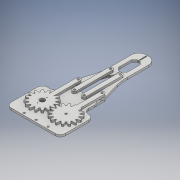
# Autodesk Inventor part: gripper_v3
Saved by Autodesk Inventor 2017 (Build 210142000, 142)
## iProperties
Created: 2016-09-29
Part Number: gripper_v3
Material: Generic
Document SubType Name: Modeling
Designer: mills
Density: 1 g/cm^3
Appearance: Default
Author: mills
Autodesk Inventor part; units mm, degrees
note: some values were not read from the file. Chosen so that the rebuilt part matches the saved one: sketch regions of "Left Gear".
ref_plane "YZ Plane" through (0, 0, 0) normal (1, 0, 0) x (0, 1, 0)
ref_plane "XZ Plane" through (0, 0, 0) normal (0, 1, 0) x (-1, 0, 0)
ref_plane "XY Plane" through (0, 0, 0) normal (0, 0, 1) x (1, 0, 0)
sketch "main drive" plane through (0, 0, 0) normal (0, 0, 1) x (1, 0, 0)
  arc A0 (-24.196, 16.2718) -> (-23.4404, 11.5793) centre (-9.5057, 16.2302) ccw
  arc A1 (-23.4404, 11.5793) -> (-24.5419, 10.8433) centre (-16.5, 0) ccw
  arc A2 (-24.5419, 10.8433) -> (-28.5881, 13.3371) centre (-34.1714, -0.2508) ccw
  arc A3 (-28.5881, 13.3371) -> (-29.8371, 12.0881) centre (-16.5, 0) ccw
  arc A4 (-29.8371, 12.0881) -> (-27.3433, 8.0419) centre (-16.2492, 17.6714) ccw
  arc A5 (-27.3433, 8.0419) -> (-28.0793, 6.9404) centre (-16.5, 0) ccw
  arc A6 (-28.0793, 6.9404) -> (-32.7718, 7.696) centre (-32.7302, -6.9943) ccw
  arc A7 (-32.7718, 7.696) -> (-33.4478, 6.064) centre (-16.5, 0) ccw
  arc A8 (-33.4478, 6.064) -> (-29.5954, 3.2802) centre (-23.0308, 16.4222) ccw
  arc A9 (-29.5954, 3.2802) -> (-29.8539, 1.9809) centre (-16.5, 0) ccw
  arc A10 (-29.8539, 1.9809) -> (-34.4783, 0.8832) centre (-28.8182, -12.6729) ccw
  arc A11 (-34.4783, 0.8832) -> (-34.4783, -0.8832) centre (-16.5, 0) ccw
  arc A12 (-34.4783, -0.8832) -> (-29.8539, -1.9809) centre (-28.8182, 12.6729) ccw
  arc A13 (-29.8539, -1.9809) -> (-29.5954, -3.2802) centre (-16.5, 0) ccw
  arc A14 (-29.5954, -3.2802) -> (-33.4478, -6.064) centre (-23.0308, -16.4222) ccw
  arc A15 (-33.4478, -6.064) -> (-32.7718, -7.696) centre (-16.5, 0) ccw
  arc A16 (-32.7718, -7.696) -> (-28.0793, -6.9404) centre (-32.7302, 6.9943) ccw
  arc A17 (-28.0793, -6.9404) -> (-27.3433, -8.0419) centre (-16.5, 0) ccw
  arc A18 (-27.3433, -8.0419) -> (-29.8371, -12.0881) centre (-16.2492, -17.6714) ccw
  arc A19 (-29.8371, -12.0881) -> (-28.5881, -13.3371) centre (-16.5, 0) ccw
  arc A20 (-28.5881, -13.3371) -> (-24.5419, -10.8433) centre (-34.1714, 0.2508) ccw
  arc A21 (-24.5419, -10.8433) -> (-23.4404, -11.5793) centre (-16.5, 0) ccw
  arc A22 (-23.4404, -11.5793) -> (-24.196, -16.2718) centre (-9.5057, -16.2302) ccw
  arc A23 (-24.196, -16.2718) -> (-22.564, -16.9478) centre (-16.5, 0) ccw
  arc A24 (-22.564, -16.9478) -> (-19.7802, -13.0954) centre (-32.9222, -6.5308) ccw
  arc A25 (-19.7802, -13.0954) -> (-18.4809, -13.3539) centre (-16.5, 0) ccw
  arc A26 (-18.4809, -13.3539) -> (-17.3832, -17.9783) centre (-3.8271, -12.3182) ccw
  arc A27 (-17.3832, -17.9783) -> (-15.6168, -17.9783) centre (-16.5, 0) ccw
  arc A28 (-15.6168, -17.9783) -> (-14.5191, -13.3539) centre (-29.1729, -12.3182) ccw
  arc A29 (-14.5191, -13.3539) -> (-13.2198, -13.0954) centre (-16.5, 0) ccw
  arc A30 (-13.2198, -13.0954) -> (-10.436, -16.9478) centre (-0.0778, -6.5308) ccw
  arc A31 (-10.436, -16.9478) -> (-8.804, -16.2718) centre (-16.5, 0) ccw
  arc A32 (-8.804, -16.2718) -> (-9.5596, -11.5793) centre (-23.4943, -16.2302) ccw
  arc A33 (-9.5596, -11.5793) -> (-8.4581, -10.8433) centre (-16.5, 0) ccw
  arc A34 (-8.4581, -10.8433) -> (-4.4119, -13.3371) centre (1.1714, 0.2508) ccw
  arc A35 (-4.4119, -13.3371) -> (-3.1629, -12.0881) centre (-16.5, 0) ccw
  arc A36 (-3.1629, -12.0881) -> (-5.6567, -8.0419) centre (-16.7508, -17.6714) ccw
  arc A37 (-5.6567, -8.0419) -> (-4.9207, -6.9404) centre (-16.5, 0) ccw
  arc A38 (-4.9207, -6.9404) -> (-0.2282, -7.696) centre (-0.2698, 6.9943) ccw
  arc A39 (-0.2282, -7.696) -> (0.4478, -6.064) centre (-16.5, 0) ccw
  arc A40 (0.4478, -6.064) -> (-3.4046, -3.2802) centre (-9.9692, -16.4222) ccw
  arc A41 (-3.4046, -3.2802) -> (-3.1461, -1.9809) centre (-16.5, 0) ccw
  arc A42 (-3.1461, -1.9809) -> (1.4783, -0.8832) centre (-4.1818, 12.6729) ccw
  arc A43 (1.4783, -0.8832) -> (1.4783, 0.8832) centre (-16.5, 0) ccw
  arc A44 (1.4783, 0.8832) -> (-3.1461, 1.9809) centre (-4.1818, -12.6729) ccw
  arc A45 (-3.1461, 1.9809) -> (-3.4046, 3.2802) centre (-16.5, 0) ccw
  arc A46 (-3.4046, 3.2802) -> (0.4478, 6.064) centre (-9.9692, 16.4222) ccw
  arc A47 (0.4478, 6.064) -> (-0.2282, 7.696) centre (-16.5, 0) ccw
  arc A48 (-0.2282, 7.696) -> (-4.9207, 6.9404) centre (-0.2698, -6.9943) ccw
  arc A49 (-4.9207, 6.9404) -> (-5.6567, 8.0419) centre (-16.5, 0) ccw
  arc A50 (-5.6567, 8.0419) -> (-3.1629, 12.0881) centre (-16.7508, 17.6714) ccw
  arc A51 (-3.1629, 12.0881) -> (-4.4119, 13.3371) centre (-16.5, 0) ccw
  arc A52 (-4.4119, 13.3371) -> (-8.4581, 10.8433) centre (1.1714, -0.2508) ccw
  arc A53 (-8.4581, 10.8433) -> (-9.5596, 11.5793) centre (-16.5, 0) ccw
  arc A54 (-9.5596, 11.5793) -> (-8.804, 16.2718) centre (-23.4943, 16.2302) ccw
  arc A55 (-8.804, 16.2718) -> (-10.436, 16.9478) centre (-16.5, 0) ccw
  arc A56 (-10.436, 16.9478) -> (-13.2198, 13.0954) centre (-0.0778, 6.5308) ccw
  arc A57 (-13.2198, 13.0954) -> (-14.5191, 13.3539) centre (-16.5, 0) ccw
  arc A58 (-14.5191, 13.3539) -> (-15.6168, 17.9783) centre (-29.1729, 12.3182) ccw
  arc A59 (-15.6168, 17.9783) -> (-17.3832, 17.9783) centre (-16.5, 0) ccw
  arc A60 (-17.3832, 17.9783) -> (-18.4809, 13.3539) centre (-3.8271, 12.3182) ccw
  arc A61 (-18.4809, 13.3539) -> (-19.7802, 13.0954) centre (-16.5, 0) ccw
  arc A62 (-19.7802, 13.0954) -> (-22.564, 16.9478) centre (-32.9222, 6.5308) ccw
  arc A63 (-22.564, 16.9478) -> (-24.196, 16.2718) centre (-16.5, 0) ccw
  arc A64 (5.8406, 14.5044) -> (7.4777, 10.0423) centre (20.2689, 17.2666) ccw
  arc A65 (7.4777, 10.0423) -> (6.5368, 9.1096) centre (16.5, 0) ccw
  arc A66 (6.5368, 9.1096) -> (2.0892, 10.7856) centre (-0.7989, -3.6181) ccw
  arc A67 (2.0892, 10.7856) -> (1.1014, 9.3211) centre (16.5, 0) ccw
  arc A68 (1.1014, 9.3211) -> (4.3214, 5.8252) centre (13.3744, 17.3946) ccw
  arc A69 (4.3214, 5.8252) -> (3.8091, 4.6034) centre (16.5, 0) ccw
  arc A70 (3.8091, 4.6034) -> (-0.9413, 4.4498) centre (1.9025, -9.9627) ccw
  arc A71 (-0.9413, 4.4498) -> (-1.2935, 2.7188) centre (16.5, 0) ccw
  arc A72 (-1.2935, 2.7188) -> (3.0193, 0.7212) centre (6.9557, 14.8744) ccw
  arc A73 (3.0193, 0.7212) -> (3.0135, -0.6036) centre (16.5, 0) ccw
  arc A74 (3.0135, -0.6036) -> (-1.3165, -2.5634) centre (6.8262, -14.7905) ccw
  arc A75 (-1.3165, -2.5634) -> (-0.9795, -4.2974) centre (16.5, 0) ccw
  arc A76 (-0.9795, -4.2974) -> (3.7694, -4.4925) centre (1.99, 10.0897) ccw
  arc A77 (3.7694, -4.4925) -> (4.2711, -5.7187) centre (16.5, 0) ccw
  arc A78 (4.2711, -5.7187) -> (1.0206, -9.1864) centre (13.2227, -17.3666) ccw
  arc A79 (1.0206, -9.1864) -> (1.9956, -10.6594) centre (16.5, 0) ccw
  arc A80 (1.9956, -10.6594) -> (6.4577, -9.0223) centre (-0.7666, 3.7689) ccw
  arc A81 (6.4577, -9.0223) -> (7.3904, -9.9632) centre (16.5, 0) ccw
  arc A82 (7.3904, -9.9632) -> (5.7144, -14.4108) centre (20.1181, -17.2988) ccw
  arc A83 (5.7144, -14.4108) -> (7.1789, -15.3986) centre (16.5, 0) ccw
  arc A84 (7.1789, -15.3986) -> (10.6748, -12.1786) centre (-0.8946, -3.1256) ccw
  arc A85 (10.6748, -12.1786) -> (11.8966, -12.6909) centre (16.5, 0) ccw
  arc A86 (11.8966, -12.6909) -> (12.0502, -17.4413) centre (26.4627, -14.5975) ccw
  arc A87 (12.0502, -17.4413) -> (13.7812, -17.7935) centre (16.5, 0) ccw
  arc A88 (13.7812, -17.7935) -> (15.7788, -13.4807) centre (1.6256, -9.5443) ccw
  arc A89 (15.7788, -13.4807) -> (17.1036, -13.4865) centre (16.5, 0) ccw
  arc A90 (17.1036, -13.4865) -> (19.0634, -17.8165) centre (31.2905, -9.6737) ccw
  arc A91 (19.0634, -17.8165) -> (20.7974, -17.4795) centre (16.5, 0) ccw
  arc A92 (20.7974, -17.4795) -> (20.9925, -12.7306) centre (6.4103, -14.51) ccw
  arc A93 (20.9925, -12.7306) -> (22.2187, -12.2289) centre (16.5, 0) ccw
  arc A94 (22.2187, -12.2289) -> (25.6864, -15.4793) centre (33.8666, -3.2773) ccw
  arc A95 (25.6864, -15.4793) -> (27.1594, -14.5044) centre (16.5, 0) ccw
  arc A96 (27.1594, -14.5044) -> (25.5223, -10.0423) centre (12.7311, -17.2666) ccw
  arc A97 (25.5223, -10.0423) -> (26.4632, -9.1096) centre (16.5, 0) ccw
  arc A98 (26.4632, -9.1096) -> (30.9108, -10.7856) centre (33.7988, 3.6181) ccw
  arc A99 (30.9108, -10.7856) -> (31.8986, -9.3211) centre (16.5, 0) ccw
  arc A100 (31.8986, -9.3211) -> (28.6786, -5.8252) centre (19.6256, -17.3946) ccw
  arc A101 (28.6786, -5.8252) -> (29.1909, -4.6034) centre (16.5, 0) ccw
  arc A102 (29.1909, -4.6034) -> (33.9413, -4.4498) centre (31.0975, 9.9627) ccw
  arc A103 (33.9413, -4.4498) -> (34.2935, -2.7188) centre (16.5, 0) ccw
  arc A104 (34.2935, -2.7188) -> (29.9807, -0.7212) centre (26.0443, -14.8744) ccw
  arc A105 (29.9807, -0.7212) -> (29.9865, 0.6036) centre (16.5, 0) ccw
  arc A106 (29.9865, 0.6036) -> (34.3165, 2.5634) centre (26.1738, 14.7905) ccw
  arc A107 (34.3165, 2.5634) -> (33.9795, 4.2974) centre (16.5, 0) ccw
  arc A108 (33.9795, 4.2974) -> (29.2306, 4.4925) centre (31.01, -10.0897) ccw
  arc A109 (29.2306, 4.4925) -> (28.7289, 5.7187) centre (16.5, 0) ccw
  arc A110 (28.7289, 5.7187) -> (31.9794, 9.1864) centre (19.7773, 17.3666) ccw
  arc A111 (31.9794, 9.1864) -> (31.0044, 10.6594) centre (16.5, 0) ccw
  arc A112 (31.0044, 10.6594) -> (26.5423, 9.0223) centre (33.7666, -3.7689) ccw
  arc A113 (26.5423, 9.0223) -> (25.6096, 9.9632) centre (16.5, 0) ccw
  arc A114 (25.6096, 9.9632) -> (27.2856, 14.4108) centre (12.8819, 17.2989) ccw
  arc A115 (27.2856, 14.4108) -> (25.8211, 15.3986) centre (16.5, 0) ccw
  arc A116 (25.8211, 15.3986) -> (22.3252, 12.1786) centre (33.8946, 3.1256) ccw
  arc A117 (22.3252, 12.1786) -> (21.1034, 12.6909) centre (16.5, 0) ccw
  arc A118 (21.1034, 12.6909) -> (20.9498, 17.4413) centre (6.5373, 14.5975) ccw
  arc A119 (20.9498, 17.4413) -> (19.2188, 17.7935) centre (16.5, 0) ccw
  arc A120 (19.2188, 17.7935) -> (17.2212, 13.4807) centre (31.3744, 9.5443) ccw
  arc A121 (17.2212, 13.4807) -> (15.8964, 13.4865) centre (16.5, 0) ccw
  arc A122 (15.8964, 13.4865) -> (13.9366, 17.8165) centre (1.7095, 9.6738) ccw
  arc A123 (13.9366, 17.8165) -> (12.2026, 17.4795) centre (16.5, 0) ccw
  arc A124 (12.2026, 17.4795) -> (12.0075, 12.7306) centre (26.5897, 14.51) ccw
  arc A125 (12.0075, 12.7306) -> (10.7813, 12.2289) centre (16.5, 0) ccw
  arc A126 (10.7813, 12.2289) -> (7.3136, 15.4794) centre (-0.8666, 3.2773) ccw
  arc A127 (7.3136, 15.4794) -> (5.8406, 14.5044) centre (16.5, 0) ccw
  circle A128 centre (16.5, 0) radius 1.375
  circle A129 centre (-16.5, 6.5) radius 0.5
  circle A130 centre (-16.5, -6.5) radius 0.5
  line L0 (-16.5, 111.9513) -> (-16.5, -38.0487) construction
  line L1 (16.5, 111.9513) -> (16.5, -38.0487) construction
  line L2 (19.5, 50) -> (19.5, 0)
  line L3 (13.5, 0) -> (13.5, 50)
  circle A131 centre (16.5, 50) radius 1.375
  circle A132 centre (16.5, 50) radius 3
  line L4 (13.5, 50) -> (15.125, 50)
  line L5 (17.875, 50) -> (19.5, 50)
  line L6 (19.5, 0) -> (17.875, 0)
  line L7 (15.125, 0) -> (13.5, 0)
  line L8 (-48.3069, 0) -> (48.1802, 0) projected
  line L9 (-3.75, 85) -> (-3.75, 35)
  line L10 (-9.75, 35) -> (-9.75, 85)
  line L11 (9.75, 85) -> (9.75, 35)
  line L12 (3.75, 35) -> (3.75, 85)
  line L13 (-6.75, 111.9513) -> (-6.75, -38.0487) construction
  line L14 (6.75, 111.9513) -> (6.75, -38.0487) construction
  line L15 (0, -68.0487) -> (0, 141.9513) projected
  line L16 (-19.5, 0) -> (-13.5, 0)
  line L17 (-13.5, 0) -> (-13.5, 50)
  line L18 (-19.5, 50) -> (-19.5, 0)
  circle A133 centre (-16.5, 50) radius 3
  circle A134 centre (-16.5, 0) radius 3.45
  circle A135 centre (-16.5, 50) radius 1.375
  line L19 (-13.5, 50) -> (-15.125, 50)
  line L20 (-17.875, 50) -> (-19.5, 50)
  circle A136 centre (-6.75, 85) radius 3
  circle A137 centre (6.75, 85) radius 3
  circle A138 centre (6.75, 35) radius 3
  circle A139 centre (-6.75, 35) radius 3
  circle A140 centre (-6.75, 35) radius 1.375
  circle A141 centre (6.75, 35) radius 1.375
  circle A142 centre (6.75, 85) radius 1.375
  circle A143 centre (-6.75, 85) radius 1.375
  line L21 (-3.75, 35) -> (-5.375, 35)
  line L22 (-8.125, 35) -> (-9.75, 35)
  line L23 (9.75, 35) -> (8.125, 35)
  line L24 (5.375, 35) -> (3.75, 35)
  line L25 (3.75, 85) -> (5.375, 85)
  line L26 (8.125, 85) -> (9.75, 85)
  line L27 (-9.75, 85) -> (-8.125, 85)
  line L28 (-5.375, 85) -> (-3.75, 85)
  point P0 (0, 0)
  dimension "d15" = 2.75
  dimension "d12" = 16.5
  dimension "d13" = 16.5
  dimension "d16" = 1
  dimension "d17" = 1
  dimension "d18" = 13
  dimension "d31" = 50
  dimension "d35" = 6
  dimension "d36" = 6
  dimension "d37" = 3
  dimension "d38" = 3
  dimension "d44" = 3.75
  dimension "d46" = 3.75
  dimension "d47" = 50
  dimension "d50" = 6.5
  dimension "d51" = 50
  dimension "d52" = 6
  dimension "d53" = 6
  dimension "d54" = 3
  dimension "d55" = 3
  dimension "d56" = 6.9
  dimension "d57" = 2.75
  dimension "d58" = 2.75
  dimension "d63" = 2.75
  dimension "d64" = 2.75
  dimension "d65" = 2.75
  dimension "d66" = 2.75
  constraints: 140 point on circle, 73 centre point, 62 equal radius, 54 end point, 18 parallel, 9 horizontal alignment, 8 point on line, 8 vertical, 7 horizontal, 7 perpendicular, 6 coincident, 2 collinear, 2 vertical alignment, 203 other
  measures "d16" diameter of A129
  measures "d17" diameter of A130
  measures "d18" distance of A130.centre A129.centre
  measures "d31" distance of L2.start L2.end
  measures "d35" distance of L10.end L9.start
  measures "d36" distance of L12.end L11.start
  measures "d37" distance between parallel lines of L13 L10
  measures "d38" distance between parallel lines of L14 L11
  measures "d44" distance between parallel lines of L15 L9
  measures "d46" distance between parallel lines of L12 L15
  measures "d47" distance of L11.start L11.end
  measures "d51" distance of L18.start L16.start
  measures "d52" distance of L17.end L18.start
  measures "d53" distance between parallel lines of L2 L3
  measures "d54" distance between parallel lines of L3 L1
  measures "d55" distance between parallel lines of L17 L0
  measures "d56" diameter of A134
  measures "d57" diameter of A135
  measures "d58" diameter of A131
  measures "d63" diameter of A143
  measures "d64" diameter of A140
  measures "d65" diameter of A141
  measures "d66" diameter of A142
extrude "Left Gear" add sketch "main drive" along normal blind 3 contours A63 A62 A61 L18 A134 L8 A11 A10 A9 A8 A7 A6 A5 A4 A3 A2 A1 A0 | L18 A133 L17 A57 A58 A59 A60 A61 | A61 A60 A59 A58 A57 L17 A134 L18 | L20 A135 L19 A133 | A133 L19 A135 L20 | L17 A57 A56 A55 A54 A53 A52 A51 A50 A49 A48 A47 L15 A46 A45 A44 L8 A134 | A134 L8 L15 A42 A41 A40 A39 A38 A37 A36 A35 A34 A33 A32 A31 A30 A29 A28 A27 A26 A25 A24 A23 A22 A21 A20 A19 A18 A17 A16 A15 A14 A13 A12 A11 | L15 A44 A43 L8 | L8 A43 A42 L15 | A40 A39 L15 | L15 A47 A46
extrude "Left Gear cutout" cut sketch "main drive" along normal blind 3 contours A134 L17 L8 L18 | L18 L8 A134 | L8 A134 | A134 L8 L17
extrude "Right Gear" add sketch "main drive" along normal blind 3 separate body contours L8 L7 A128 L6 A105 A104 A103 A102 A101 A100 A99 A98 A97 A96 A95 A94 A93 A92 A91 A90 A89 A88 A87 A86 A85 A84 A83 A82 A81 A80 A79 A78 A77 A76 L15 A74 A73 | A73 A72 L15 A70 A69 A68 A67 A66 A65 A64 A127 A126 A125 A124 A123 L3 L8 | L15 A76 A75 A74 | A72 A71 A70 L15 | L3 A123 A122 A121 A120 A119 L2 L6 A128 L7 | L3 A132 L2 A119 A120 A121 A122 A123 | L4 A131 L5 A132 | A132 L5 A131 L4 | L2 A119 A118 A117 A116 A115 A114 A113 A112 A111 A110 A109 A108 A107 A106 A105 L8
extrude "Left Strut" add sketch "main drive" along normal blind 3 separate body contours L28 A143 L27 A136 | L9 A139 L10 A136 | A136 L27 A143 L28 | L21 A140 L22 A139 | A139 L22 A140 L21
extrude "Right Strut" add sketch "main drive" along normal blind 3 separate body contours L26 A142 L25 A137 | L11 A138 L12 A137 | A137 L25 A142 L26 | L23 A141 L24 A138 | A138 L24 A141 L23
sketch "grip + base" plane through (0, 0, 0) normal (0, 0, -1) x (-1, 0, 0)
  line L0 (4.0208, 79.5) -> (12.0208, 79.5)
  line L1 (12.0208, 89.186) -> (12.0208, 119.3579)
  line L2 (1.8786, 129.5) -> (0.0208, 129.5)
  line L3 (0.0208, 129.5) -> (0.0208, 83.5)
  line L4 (0.0208, 117.5) -> (2.0208, 117.5)
  line L5 (6.0208, 113.5) -> (6.0208, 95.5)
  line L6 (2.0208, 91.5) -> (0.0208, 91.5)
  line L7 (0.0208, 91.5) -> (0.0208, 117.5)
  line L8 (2.0208, 117.5) -> (6.0208, 113.5)
  line L9 (6.0208, 95.5) -> (2.0208, 91.5)
  line L10 (8.9497, 126.5711) -> (9.0918, 126.4289)
  line L11 (0.0208, 128.2) -> (0.8868, 127.7)
  line L12 (0.8868, 127.7) -> (0.0208, 127.2)
  line L13 (0.0208, 128.2) -> (0.0208, 127.2)
  line L14 (0.0208, 127) -> (0.8868, 126.5)
  line L15 (0.0208, 127) -> (0.0208, 126)
  line L16 (0.8868, 126.5) -> (0.0208, 126)
  line L17 (0.0208, 125.8) -> (0.8868, 125.3)
  line L18 (0.0208, 125.8) -> (0.0208, 124.8)
  line L19 (0.8868, 125.3) -> (0.0208, 124.8)
  line L20 (0.0208, 124.6) -> (0.8868, 124.1)
  line L21 (0.0208, 124.6) -> (0.0208, 123.6)
  line L22 (0.8868, 124.1) -> (0.0208, 123.6)
  line L23 (0.0208, 123.4) -> (0.8868, 122.9)
  line L24 (0.0208, 123.4) -> (0.0208, 122.4)
  line L25 (0.8868, 122.9) -> (0.0208, 122.4)
  line L26 (0.0208, 122.2) -> (0.8868, 121.7)
  line L27 (0.0208, 122.2) -> (0.0208, 121.2)
  line L28 (0.8868, 121.7) -> (0.0208, 121.2)
  line L29 (0.0208, 121) -> (0.8868, 120.5)
  line L30 (0.0208, 121) -> (0.0208, 120)
  line L31 (0.8868, 120.5) -> (0.0208, 120)
  line L32 (0.0208, 119.8) -> (0.8868, 119.3)
  line L33 (0.0208, 119.8) -> (0.0208, 118.8)
  line L34 (0.8868, 119.3) -> (0.0208, 118.8)
  line L35 (6.75, 85) -> (16.5, 50) construction
  line L36 (4.7706, 77.1999) -> (12.6467, 48.9266)
  line L37 (20.3533, 51.0734) -> (14.2215, 73.0848)
  arc A0 (10.6033, 86.0734) -> (2.8967, 83.9266) centre (6.75, 85) ccw
  arc A1 (12.6467, 48.9266) -> (20.3533, 51.0734) centre (16.5, 50) ccw
  arc A2 (12.0208, 89.186) -> (14.2215, 73.0848) centre (72.0208, 89.186) ccw
  arc A3 (12.0208, 119.3579) -> (9.0918, 126.4289) centre (2.0208, 119.3579) ccw
  arc A4 (8.9497, 126.5711) -> (1.8786, 129.5) centre (1.8786, 119.5) ccw
  line L38 (12.0208, 79.5) -> (12.8078, 79.5)
  arc A5 (0.0208, 83.5) -> (2.469, 79.8133) centre (4.0208, 83.5) ccw
  arc A6 (4.7706, 77.1999) -> (2.469, 79.8133) centre (0.9173, 76.1265) ccw
  circle A7 centre (6.75, 85) radius 1.375 projected
  circle A8 centre (16.5, 50) radius 1.375 projected
  line L39 (0, -47.6407) -> (0, 159.8439) projected
  line L40 (-4.0208, 79.5) -> (-12.0208, 79.5)
  line L41 (-12.0208, 89.186) -> (-12.0208, 119.3579)
  line L42 (-1.8786, 129.5) -> (-0.0208, 129.5)
  line L43 (-0.0208, 129.5) -> (-0.0208, 83.5)
  line L44 (-0.0208, 117.5) -> (-2.0208, 117.5)
  line L45 (-6.0208, 113.5) -> (-6.0208, 95.5)
  line L46 (-2.0208, 91.5) -> (-0.0208, 91.5)
  line L47 (-0.0208, 91.5) -> (-0.0208, 117.5)
  line L48 (-2.0208, 117.5) -> (-6.0208, 113.5)
  line L49 (-6.0208, 95.5) -> (-2.0208, 91.5)
  line L50 (-8.9497, 126.5711) -> (-9.0918, 126.4289)
  line L51 (-0.0208, 128.2) -> (-0.8868, 127.7)
  line L52 (-0.8868, 127.7) -> (-0.0208, 127.2)
  line L53 (-0.0208, 128.2) -> (-0.0208, 127.2)
  line L54 (-0.0208, 127) -> (-0.8868, 126.5)
  line L55 (-0.0208, 127) -> (-0.0208, 126)
  line L56 (-0.8868, 126.5) -> (-0.0208, 126)
  line L57 (-0.0208, 125.8) -> (-0.8868, 125.3)
  line L58 (-0.0208, 125.8) -> (-0.0208, 124.8)
  line L59 (-0.8868, 125.3) -> (-0.0208, 124.8)
  line L60 (-0.0208, 124.6) -> (-0.8868, 124.1)
  line L61 (-0.0208, 124.6) -> (-0.0208, 123.6)
  line L62 (-0.8868, 124.1) -> (-0.0208, 123.6)
  line L63 (-0.0208, 123.4) -> (-0.8868, 122.9)
  line L64 (-0.0208, 123.4) -> (-0.0208, 122.4)
  line L65 (-0.8868, 122.9) -> (-0.0208, 122.4)
  line L66 (-0.0208, 122.2) -> (-0.8868, 121.7)
  line L67 (-0.0208, 122.2) -> (-0.0208, 121.2)
  line L68 (-0.8868, 121.7) -> (-0.0208, 121.2)
  line L69 (-0.0208, 121) -> (-0.8868, 120.5)
  line L70 (-0.0208, 121) -> (-0.0208, 120)
  line L71 (-0.8868, 120.5) -> (-0.0208, 120)
  line L72 (-0.0208, 119.8) -> (-0.8868, 119.3)
  line L73 (-0.0208, 119.8) -> (-0.0208, 118.8)
  line L74 (-0.8868, 119.3) -> (-0.0208, 118.8)
  line L75 (-6.75, 85) -> (-16.5, 50) construction
  line L76 (-4.7706, 77.1999) -> (-12.6467, 48.9266)
  line L77 (-20.3533, 51.0734) -> (-14.2215, 73.0848)
  arc A9 (-2.8967, 83.9266) -> (-10.6033, 86.0734) centre (-6.75, 85) ccw
  arc A10 (-20.3533, 51.0734) -> (-12.6467, 48.9266) centre (-16.5, 50) ccw
  arc A11 (-14.2215, 73.0848) -> (-12.0208, 89.186) centre (-72.0208, 89.186) ccw
  arc A12 (-9.0918, 126.4289) -> (-12.0208, 119.3579) centre (-2.0208, 119.3579) ccw
  arc A13 (-1.8786, 129.5) -> (-8.9497, 126.5711) centre (-1.8786, 119.5) ccw
  line L78 (-12.0208, 79.5) -> (-12.8078, 79.5)
  arc A14 (-2.469, 79.8133) -> (-0.0208, 83.5) centre (-4.0208, 83.5) ccw
  arc A15 (-2.469, 79.8133) -> (-4.7706, 77.1999) centre (-0.9173, 76.1265) ccw
  circle A16 centre (-6.75, 85) radius 1.375
  circle A17 centre (-16.5, 50) radius 1.375
  point P0 (0, 0)
  point P1 (12.0208, 129.5)
  point P2 (-6.75, 85)
  point P3 (6.0208, 91.5)
  point P4 (6.0208, 117.5)
  point P5 (6.0208, 129.5)
  point P6 (12.0208, 123.5)
  point P7 (-16.5, 50)
  point P8 (11.625, 67.5)
  point P9 (-12.0208, 129.5)
  point P10 (6.75, 85)
  point P11 (-6.0208, 91.5)
  point P12 (-6.0208, 117.5)
  point P13 (-6.0208, 129.5)
  point P14 (-12.0208, 123.5)
  point P15 (16.5, 50)
  point P16 (-11.625, 67.5)
  dimension "d73" = 12
  dimension "d74" = 50
  dimension "d75" = 5.5
  dimension "d76" = 6
  dimension "d77" = 12
  dimension "d78" = 12
  dimension "d79" = 4
  dimension "d80" = 4
  dimension "d81" = 4
  dimension "d82" = 4
  dimension "d83" = 6
  dimension "d84" = 6
  dimension "d86" = 1
  dimension "d87" = 1
  dimension "d88" = 1
  dimension "d91" = 1.2
  dimension "d96" = 1.3
  dimension "d97" = 9.4
  dimension "d98" = 8
  dimension "d99" = 60
  dimension "d100" = 10
  dimension "d101" = 10
  dimension "d102" = 4
  dimension "d103" = 4
  constraints: 160 end point, 64 symmetric about line, 32 point on circle, 32 point on line, 16 centre point, 14 tangent, 5 parallel, 3 horizontal, 2 perpendicular, 1 collinear, 1 midpoint, 1 vertical, 51 other
  measures "d73" distance of point (12.021, 129.5) L2.end
  measures "d74" distance of L0.end point (12.021, 129.5)
  measures "d75" distance from line of L0 L35.start
  measures "d76" distance of L4.start point (6.021, 117.5)
  measures "d77" distance between parallel lines of L4 L2
  measures "d78" distance between parallel lines of L6 L0
  measures "d79" distance of L4.end point (6.021, 117.5)
  measures "d80" distance of L5.start point (6.021, 117.5)
  measures "d81" distance of L5.end point (6.021, 91.5)
  measures "d82" distance of L6.start point (6.021, 91.5)
  measures "d83" distance of point (6.021, 129.5) point (12.021, 129.5)
  measures "d84" distance of point (12.021, 123.5) point (12.021, 129.5)
  measures "d86" distance of L11.end L12.end
  measures "d87" distance of L11.start L11.end
  measures "d88" distance of L12.end L11.start
  measures "d91" distance of L11.start L14.start
  measures "d96" distance of L2.end L11.start
  measures "d97" distance of L33.end L11.start
  measures "d98" distance between parallel lines of L37 L36
  measures "d99" radius of A2
  measures "d100" radius of A3
  measures "d101" radius of A4
  measures "d102" radius of A5
  measures "d103" radius of A6
extrude "Left Clamp" add sketch "grip + base" along normal blind 3 separate body contours A2 L37 A1 L36 A6 A5 L3 L6 L9 L5 L8 L4 L34 L32 L31 L29 L28 L26 L25 L23 L22 L20 L19 L17 L16 L14 L12 L11 L2 A4 L10 A3 L1
extrude "Right Clamp" add sketch "grip + base" along normal blind 3 separate body contours L41 A12 L50 A13 L42 L43 L51 L52 L54 L56 L57 L59 L60 L62 L63 L65 L66 L68 L69 L71 L72 L74 L44 L48 L45 L49 L46 A14 A15 L76 A10 L77 A11
sketch "Base Sktch" plane through (0, 0, 0) normal (0, 0, -1) x (-1, 0, 0)
  line L0 (13.5, 40) -> (-15.5, 40)
  line L1 (-36.5115, 11) -> (-36.5115, -21)
  line L2 (-29.5115, -28) -> (31.4938, -28)
  line L3 (38.4938, -21) -> (38.4938, 15)
  line L4 (16.5, 111.9513) -> (16.5, -38.0487) construction
  line L5 (-16.5, 111.9513) -> (-16.5, -38.0487) construction
  arc A0 (20.5, 33) -> (13.5, 40) centre (13.5, 33) ccw
  arc A1 (-15.5, 40) -> (-22.5, 33) centre (-15.5, 33) ccw
  line L6 (48.3069, 0) -> (-48.1802, 0) projected
  line L7 (31.4938, 22) -> (27.5, 22)
  line L8 (-29.5, 18) -> (-29.5115, 18)
  line L9 (20.5, 29) -> (20.5, 33)
  line L10 (-22.5, 33) -> (-22.5, 25)
  arc A2 (20.5, 29) -> (27.5, 22) centre (27.5, 29) ccw
  arc A3 (38.4938, 15) -> (31.4938, 22) centre (31.4938, 15) ccw
  arc A4 (-29.5, 18) -> (-22.5, 25) centre (-29.5, 25) ccw
  arc A5 (-29.5115, 18) -> (-36.5115, 11) centre (-29.5115, 11) ccw
  line L11 (22.375, 16.6) -> (10.625, 16.6)
  line L12 (10.625, 16.6) -> (10.625, -5.8)
  line L13 (10.625, -5.8) -> (22.375, -5.8)
  line L14 (22.375, -5.8) -> (22.375, 16.6)
  line L15 (7.625, 21.6) -> (25.375, 21.6)
  line L16 (25.375, 21.6) -> (25.375, -10.8)
  line L17 (25.375, -10.8) -> (7.625, -10.8)
  line L18 (7.625, -10.8) -> (7.625, 21.6)
  circle A6 centre (16.5, 18.85) radius 1
  circle A7 centre (16.5, -8.05) radius 1
  circle A8 centre (-16.5, -25) radius 1.375
  circle A9 centre (0, -25) radius 1.375
  circle A10 centre (16.5, -25) radius 1.375
  arc A11 (-36.5115, -21) -> (-29.5115, -28) centre (-29.5115, -21) ccw
  arc A12 (31.4938, -28) -> (38.4938, -21) centre (31.4938, -21) ccw
  circle A13 centre (-16.5, 0) radius 1.375 projected
  circle A14 centre (-6.75, 35) radius 1.375 projected
  circle A15 centre (6.75, 35) radius 1.375 projected
  point P0 (0, 0)
  point P1 (16.5, 22)
  point P2 (-16.5, 18)
  point P3 (20.5, 0)
  point P4 (-22.5, 0)
  point P5 (16.5, 0)
  dimension "d116" = 5
  dimension "d119" = 7
  dimension "d122" = 28
  dimension "d123" = 7
  dimension "d125" = 11.75
  dimension "d126" = 22.4
  dimension "d128" = 5.875
  dimension "d129" = 17.75
  dimension "d130" = 32.4
  dimension "d133" = 8.875
  dimension "d135" = 5
  dimension "d136" = 2
  dimension "d137" = 2
  dimension "d138" = 2.25
  dimension "d139" = 2.25
  dimension "d140" = 2.75
  dimension "d141" = 2.75
  dimension "d142" = 2.75
  dimension "d143" = 3
  dimension "d144" = 3
  dimension "d145" = 3
  dimension "d146" = 7
  dimension "d161" = 5.8
  constraints: 32 end point, 16 point on circle, 16 tangent, 14 point on line, 13 centre point, 8 parallel, 5 equal radius, 5 horizontal, 5 perpendicular
  measures "d116" distance from line of L0 point (6.75, 35)
  measures "d119" radius of A0
  measures "d122" distance between parallel lines of L6 L2
  measures "d123" radius of A2
  measures "d125" distance of L12.end L13.end
  measures "d126" distance of L13.end L11.start
  measures "d128" distance from line of L14 point (16.5, 0)
  measures "d129" distance of L15.start L15.end
  measures "d130" distance of L15.end L16.end
  measures "d133" distance between parallel lines of L4 L18
  measures "d135" distance between parallel lines of L15 L11
  measures "d136" diameter of A6
  measures "d137" diameter of A7
  measures "d138" distance from line of A6.centre L11
  measures "d139" distance from line of L13 A7.centre
  measures "d140" diameter of A8
  measures "d141" diameter of A9
  measures "d142" diameter of A10
  measures "d143" distance from line of L2 A8.centre
  measures "d144" distance from line of L2 A9.centre
  measures "d145" distance from line of L2 A10.centre
  measures "d146" radius of A11
  measures "d161" distance from line of L13 point (16.5, 0)
extrude "Servo Mount" add sketch "Base Sktch" along normal blind 8 separate body contours L16 L17 L18 L6 L12 L13 L14 | L6 L14 L11 L12 L18 L15 L16
extrude "Base" add sketch "Base Sktch" along normal blind 3 contours A0 L9 A2 L7 A3 L3 L6 L16 L15 L18 A13 L1 A5 L8 A4 L10 A1 L0 | L3 A12 L2 A11 L1 L6 A13 L18 L17 L16 bodies 7
sketch "Gear Strut" plane through (0, 0, -3) normal (0, 0, -1) x (-1, 0, 0)
  circle A0 centre (-16.5, 50) radius 1.375 projected
  circle A1 centre (-16.5, 0) radius 1.375 projected
  line L0 (-16.5, 50) -> (-16.5, 0) construction
  line L1 (-13.5, 50) -> (-13.5, 0)
  line L2 (-19.5, 0) -> (-19.5, 50)
  arc A2 (-13.5, 50) -> (-19.5, 50) centre (-16.5, 50) ccw
  arc A3 (-19.5, 0) -> (-13.5, 0) centre (-16.5, 0) ccw
  circle A4 centre (-16.5, 50) radius 1.375 projected
  point P0 (0, 0)
  point P1 (-16.5, 25)
  dimension "d162" = 6
  constraints: 8 end point, 4 point on circle, 4 tangent, 2 centre point, 1 midpoint, 1 parallel, 1 vertical
  measures "d162" distance between parallel lines of L2 L1
extrude "Support Strut" add sketch "Gear Strut" along normal blind 3 separate body
equation "\"d13\" = d12"
equation "\"d31\" = d51"
equation "\"d35\" = d52"
equation "\"d36\" = d35"
equation "\"d37\" = 0.5 * d35"
equation "\"d38\" = 0.5 * d36"
equation "\"d44\" = -0.5 * d35 + 0.5 * d12 - 0.5 * d55"
equation "\"d46\" = d44"
equation "\"d47\" = d51"
equation "\"d50\" = 0.5 * d18"
equation "\"d53\" = d52"
equation "\"d54\" = 0.5 * d53"
equation "\"d55\" = 0.5 * d52"
equation "\"d58\" = d57"
equation "\"d63\" = d57"
equation "\"d64\" = d57"
equation "\"d65\" = d57"
equation "\"d66\" = d57"
equation "\"d73\" = 2 * d52"
equation "\"d74\" = d51"
equation "\"d75\" = 2 * d63"
equation "\"d76\" = 0.5 * d73"
equation "\"d77\" = d73"
equation "\"d78\" = d77"
equation "\"d80\" = d79"
equation "\"d82\" = d81"
equation "\"d83\" = d52"
equation "\"d84\" = d83"
equation "\"d22\" = 0.5 * d19"
equation "\"d19\" = 6.9"
